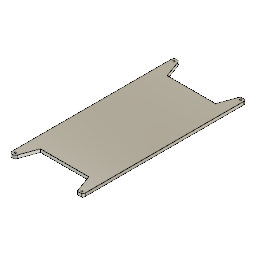
1-Heated Build Plate v1 (Autodesk Fusion 360 design; units mm, degrees)
Autodesk Fusion 360 part; units mm, degrees
mesh "Mesh1" [no effect]
sketch "Mesh Selection Sketch" plane through (0, 0, 20) normal (0, 0, 1) x (1, 0, 0)
sketch "Sketch2" plane through (0, 0, 0) normal (0, 0, 1) x (1, 0, 0)
  line L0 (-115, 260) -> (115, 260)
  line L1 (115, 260) -> (115, -260)
  line L2 (115, -260) -> (-115, -260)
  line L3 (-115, -260) -> (-115, 260)
  line L4 (-115, 260) -> (115, -260) construction
  line L5 (115, 260) -> (-115, -260) construction
  circle A0 centre (-105, 250) radius 2.75
  arc A1 (-95, 250) -> (-115, 250) centre (-105, 250) ccw
  line L6 (-105, 250) -> (-95, 250) construction
  line L7 (-105, 250) -> (-115, 250) construction
  line L8 (-95.6031, 253.4202) -> (-76.1597, 200)
  arc A2 (114.9897, 249.5472) -> (95.0071, 249.6244) centre (105, 250) ccw
  circle A3 centre (105, 250) radius 2.75
  line L9 (-76.1597, 200) -> (76.1597, 200)
  line L10 (95.6031, 253.4202) -> (76.1597, 200)
  line L11 (20, 0) -> (2.5, 0)
  circle A4 centre (105, -250) radius 2.75
  arc A5 (95.0071, -249.6244) -> (114.9897, -249.5472) centre (105, -250) ccw
  line L12 (-95.6031, -253.4202) -> (-76.1597, -200)
  line L13 (-76.1597, -200) -> (76.1597, -200)
  line L14 (95.6031, -253.4202) -> (76.1597, -200)
  arc A6 (-115, -250) -> (-95, -250) centre (-105, -250) ccw
  circle A7 centre (-105, -250) radius 2.75
  line L15 (98.3856, -257.5) -> (111.6144, -257.5)
  line L16 (98.3856, 257.5) -> (111.6144, 257.5)
  dimension "d1" = 5.5
  dimension "d2" = 10
  dimension "d3" = 10
  dimension "d4" = 180
  dimension "d5" = 60
  dimension "d7" = 230
  dimension "d8" = 520
  dimension "d9" = 10
  dimension "d10" = 10
  dimension "d11" = 110
  dimension "d14" = 7.5
  constraint horizontal L0
  constraint vertical L1
  constraint horizontal L2
  constraint vertical L3
  constraint coincident origin L5
  constraint coincident origin L4
  constraint coincident L3 A1.end
  constraint coincident A0.centre A1.centre
  constraint coincident A1 L8.start
  constraint tangent A1 L8
  constraint coincident A2 L10.start
  constraint tangent A2 L10
  constraint equal L8 L10
  constraint coincident A2.centre A3.centre
  constraint tangent L1 A2
  constraint tangent L3 A1
  constraint equal A0 A3
  constraint symmetric L8.end L11 L12.end
  constraint symmetric A0 L11 A7
  constraint symmetric A1.start L11 A6.end
  constraint symmetric A1.end L11 A6.start
  constraint symmetric A1 L11 A6
  constraint symmetric L8.start L11 L12.start
  constraint symmetric A2.end L11 A5.start
  constraint symmetric A2.start L11 A5.end
  constraint symmetric A2 L11 A5
  constraint symmetric A3 L11 A4
  constraint symmetric L9.end L11 L13.end
  constraint symmetric L10.start L11 L14.start
  constraint coincident A5 L15.start
  constraint coincident A5 L15.end
  constraint parallel L2 L15
  constraint coincident A2 L16.start
  constraint coincident A2 L16.end
  constraint parallel L0 L16
  constraint symmetric L11 L15 L16
  measures "d1" diameter of A0
  measures "d2" distance of L3 A0.centre
  measures "d3" distance of L0 A0.centre
  measures "d4" angle of L6 L7
  measures "d5" distance of L0 L9
  measures "d7" distance of L1.end L2.end
  measures "d8" distance of L0.start L2.end
  measures "d9" distance of L0 A2.centre
  measures "d10" distance of L1 A2.centre
  measures "d11" angle of L8 L9
  measures "d14" distance of A4.centre L15
extrude "Extrude1" add sketch "Sketch2" along normal blind 10 contours L1 L3 A1 L8 A2 L9 L10 A5 L12 L13 L14 A6 L15 L16
equation "d3 = d2"
equation "d9 = d2"
equation "d10 = d2"
